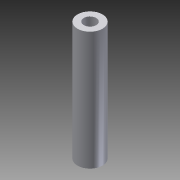
# Autodesk Inventor part: HOTENDone_PTFE
Saved by Autodesk Inventor 2015 (Build 190159000, 159)
## iProperties
Company: MARCHA TECHNOLOGY
Created: 2013-10-31
Part Number: HOTENDone_PTFE
Document SubType Name: Modeling
Designer: O.Martin
Density: 1 g/cm^3
Mass: 0.311018 g
Surface Area: 6.40885 cm^2
Volume: 0.311018 cm^3
Project: WITBOXprinter_K01
Description: TUBO PTFE HOT-END
Stock Number: 28656
Material: Generic
Appearance: Cool White
Author: O.Martin
Autodesk Inventor part; units mm, degrees
ref_plane "YZ Plane" through (0, 0, 0) normal (1, 0, 0) x (0, 1, 0)
ref_plane "XZ Plane" through (0, 0, 0) normal (0, 1, 0) x (-1, 0, 0)
ref_plane "XY Plane" through (0, 0, 0) normal (0, 0, 1) x (1, 0, 0)
sketch "Boceto1" plane through (0, 0, 0) normal (0, 0, 1) x (1, 0, 0)
  circle A0 centre (0, 0) radius 2
  circle A1 centre (0, 0) radius 1
  dimension "d0" = 2
  dimension "d1" = 4
  constraints: 2 centre point, 2 coincident
  measures "d0" diameter of A1
  measures "d1" diameter of A0
extrude "Extrusión1" add sketch "Boceto1" along normal blind 19
body "Solid1"
